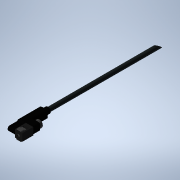
# Autodesk Inventor part: 547859 SMT-8G-PS-24V-E-2,5Q-OE_G
Saved by Autodesk Inventor 2021 (Build 250183000, 183)
## iProperties
Created: 2025-06-24
Part Number: 547859 SMT-8G-PS-24V-E-2,5Q-OE_G
Material: Generic
Catalog Web Link: www.cadenas.de
Description: SMT_G-Proximity switch
Vendor: FESTO
Document SubType Name: Modeling
Designer: psAdmin
Manufacturer: FESTO
Mass: 1.34939 g
Surface Area: 14.7047 cm^2
Volume: 1.34939 cm^3
Density: 1 g/cm^3
Appearance: PSOLRGB-51-51-51
Category: PARTsolutions
Company: FESTO
Title: 547859 SMT-8G-PS-24V-E-2,5Q-OE_G
Author: Cadenas PARTsolutions
Comments: Proximity switch
PSOL_IDENT_0: {$CADENAS_DATA/23d-libs/festo/parts/s/smt/parts/smt_g.prj},204 {VTYP=3D},{NB=547859 SMT-8G-PS-24V-E-
PSOL_IDENT_1: 2,5Q-OE_G},{LINA=547859 SMT-8G-PS-24V-E-2,5Q-OE_G},{NN=SMT_G},{DATE=12.11.2024 13:21:11},{GEOMDATE=3
PSOL_IDENT_2: 0.08.2023 07:21:55},{VERSION=},{LINEID=650},{WBVAR=},{WBNUMERIC=}  {NB=547859 SMT-8G-PS-24V-E-2,5Q-O
PSOL_IDENT_3: E_G},{LINA=547859 SMT-8G-PS-24V-E-2,5Q-OE_G},{KT=DUMMY},{TNR=547859},{TYP=SMT-8G-PS-24V-E-2,5Q-OE},{
PSOL_IDENT_4: VERS=23.000},{AT=OE},{LL=80.000}
NB: 547859 SMT-8G-PS-24V-E-2,5Q-OE_G
NN: SMT_G
NT: Proximity switch
NBSYN: $TNR. $TYP._G
LINA: 547859 SMT-8G-PS-24V-E-2,5Q-OE_G
CATALOG: Festo
TNR: 547859
TYP: SMT-8G-PS-24V-E-2,5Q-OE
VERS: 23
AT: OE
LL: 80
SUPPLIER: FESTO
ARTICLENO: 547859 SMT-8G-PS-24V-E-2,5Q-OE_G
BOMINFO: 547859 SMT-8G-PS-24V-E-2,5Q-OE_G
CREATOR: CADENAS GmbH
Autodesk Inventor part; units mm, degrees
sketch "Sketch_1" plane through (0, 0, 0) normal (0, 0, 1) x (1, 0, 0)
  arc A0 (-2.5, -2.055655) -> (-2.291667, -2.341307) centre (-2.2, -2.055655) ccw
  arc A1 (-2.291667, -2.341307) -> (2.291667, -2.341307) centre (0, 4.8) ccw
  arc A2 (2.291667, -2.341307) -> (2.5, -2.055655) centre (2.2, -2.055655) ccw
  line L0 (2.5, -2.055655) -> (2.5, 2.055655)
  arc A3 (2.5, 2.055655) -> (2.291667, 2.341307) centre (2.2, 2.055655) ccw
  arc A4 (2.291667, 2.341307) -> (-2.291667, 2.341307) centre (0, -4.8) ccw
  arc A5 (-2.291667, 2.341307) -> (-2.5, 2.055655) centre (-2.2, 2.055655) ccw
  line L1 (-2.5, 2.055655) -> (-2.5, -2.055655)
  constraints: 12 point on circle, 6 centre point, 4 end point
extrude "Extrusion1" add sketch "Sketch_1" along normal blind 22.2
sketch "Sketch_2" plane through (0, 0, 0) normal (1, 0, 0) x (0, 1, 0)
  line L0 (-3, 23.2) -> (-3, 14.3)
  line L1 (-3, 14.3) -> (-1.5, 15.8)
  line L2 (-1.5, 15.8) -> (-1.5, 21)
  arc A0 (-0.3, 22.2) -> (-1.5, 21) centre (-0.3, 21) ccw
  line L3 (-0.3, 22.2) -> (0.3, 22.2)
  arc A1 (1.5, 21) -> (0.3, 22.2) centre (0.3, 21) ccw
  line L4 (1.5, 21) -> (1.5, 15.8)
  line L5 (1.5, 15.8) -> (3, 14.3)
  line L6 (3, 14.3) -> (3, 23.2)
  line L7 (3, 23.2) -> (-3, 23.2)
  constraints: 16 end point, 4 point on circle, 2 centre point
extrude "Extrusion2" cut sketch "Sketch_2" along normal mid plane 5
sketch "Sketch_3" plane through (0, 0, 14.8) normal (0, 0, 1) x (1, 0, 0)
  line L0 (0, -2.5) -> (5, -2.5)
  arc A0 (5, -2.5) -> (7.015716, -2.224049) centre (5, 5) ccw
  arc A1 (7.015716, -2.224049) -> (7.224049, -2.015716) centre (6.935087, -1.935087) ccw
  arc A2 (7.224049, -2.015716) -> (7.224049, 2.015716) centre (0, 0) ccw
  arc A3 (7.224049, 2.015716) -> (7.015716, 2.224049) centre (6.935087, 1.935087) ccw
  arc A4 (7.015716, 2.224049) -> (5, 2.5) centre (5, -5) ccw
  line L1 (5, 2.5) -> (0, 2.5)
  line L2 (0, 2.5) -> (0, -2.5)
  constraints: 10 point on circle, 6 end point, 5 centre point
extrude "Extrusion3" add sketch "Sketch_3" against normal blind 4.8
sketch "Sketch_5" plane through (0, 0, 0) normal (0, 1, 0) x (-1, 0, 0)
  line L0 (0, -2.8) -> (0, 1)
  line L1 (0, 1) -> (2.3, 1)
  line L2 (2.3, 1) -> (2.3, 0)
  line L3 (2.3, 0) -> (2.2, 0)
  arc A0 (2.2, 0) -> (2, -0.2) centre (2.2, -0.2) ccw
  line L4 (2, -0.2) -> (2, -2.6)
  arc A1 (1.8, -2.8) -> (2, -2.6) centre (1.8, -2.6) ccw
  line L5 (1.8, -2.8) -> (0, -2.8)
  line L6 (0, -2.8) -> (0, 1)
  constraints: 14 end point, 4 point on circle, 2 centre point
revolve "Revolution1" add sketch "Sketch_5" angle 360 about axis through (0, 0, -2.8) along (0, 0, -1)
sketch "Sketch_28" plane through (0, 0, 0) normal (0, 1, 0) x (-1, 0, 0)
  circle A0 centre (0, 11.4) radius 1.55
  constraints: 1 centre point
extrude "Extrusion4" add sketch "Sketch_28" along normal mid plane 5.4
sketch "Sketch_29" plane through (0, 0, 0) normal (0, 1, 0) x (-1, 0, 0)
  circle A0 centre (0, 18.8) radius 1
  constraints: 1 centre point
extrude "Extrusion5" add sketch "Sketch_29" against normal blind 1.52
sketch "Sketch_6" plane through (0, 0, 0) normal (0, 1, 0) x (-1, 0, 0)
  line L0 (-2.5, 22.3) -> (-3.5, 22.3)
  line L1 (-3.5, 22.3) -> (-3.5, 17)
  line L2 (-3.5, 17) -> (-6.5, 17)
  line L3 (-6.5, 17) -> (-6.5, 22.3)
  line L4 (-6.5, 22.3) -> (-7.5, 22.3)
  line L5 (-7.5, 22.3) -> (-7.5, 14.8)
  line L6 (-7.5, 14.8) -> (-2.5, 14.8)
  line L7 (-2.5, 14.8) -> (-2.5, 22.3)
  constraints: 16 end point
extrude "Extrusion6" add sketch "Sketch_6" along normal mid plane 4.98
sketch "Sketch_7" plane through (5, 0, 0) normal (1, 0, 0) x (0, 0, -1)
  line L0 (-22.3, 2.95) -> (-22.3, -2.95)
  arc A0 (-22.3, -2.95) -> (-22.1, -3.15) centre (-22.1, -2.95) ccw
  line L1 (-22.1, -3.15) -> (-20, -3.15)
  arc A1 (-20, -3.15) -> (-19.8, -2.95) centre (-20, -2.95) ccw
  line L2 (-19.8, -2.95) -> (-19.8, -2.7)
  arc A2 (-19.6, -2.5) -> (-19.8, -2.7) centre (-19.6, -2.7) ccw
  line L3 (-19.6, -2.5) -> (-18.5, -2.5)
  arc A3 (-18.5, -2.5) -> (-18.3, -2.3) centre (-18.5, -2.3) ccw
  line L4 (-18.3, -2.3) -> (-18.3, 2.3)
  arc A4 (-18.3, 2.3) -> (-18.5, 2.5) centre (-18.5, 2.3) ccw
  line L5 (-18.5, 2.5) -> (-19.6, 2.5)
  arc A5 (-19.8, 2.7) -> (-19.6, 2.5) centre (-19.6, 2.7) ccw
  line L6 (-19.8, 2.7) -> (-19.8, 2.95)
  arc A6 (-19.8, 2.95) -> (-20, 3.15) centre (-20, 2.95) ccw
  line L7 (-20, 3.15) -> (-22.1, 3.15)
  arc A7 (-22.1, 3.15) -> (-22.3, 2.95) centre (-22.1, 2.95) ccw
  constraints: 16 end point, 16 point on circle, 8 centre point
extrude "Extrusion7" add sketch "Sketch_7" along normal mid plane 3
sketch "Sketch_4" plane through (0, 0, 0) normal (0, 1, 0) x (-1, 0, 0)
  line L0 (-5, 22.3) -> (-5, 10)
  line L1 (-5, 10) -> (-6.4, 10)
  line L2 (-6.4, 10) -> (-6.05, 10.35)
  line L3 (-6.05, 10.35) -> (-6.05, 18.3)
  line L4 (-6.05, 18.3) -> (-6.1, 18.3)
  line L5 (-6.1, 18.3) -> (-5.8645, 18.5355)
  line L6 (-5.8645, 18.5355) -> (-5.8645, 22.3)
  line L7 (-5.8645, 22.3) -> (-5, 22.3)
  line L8 (-5, 22.3) -> (-5, 10)
  constraints: 18 end point
revolve "Revolution2" cut sketch "Sketch_4" angle 360 about axis through (5, 0, 22.3) along (0, 0, 1)
thread "Thread1" size "M2x0.25" class "6H" standard "ISO Metric profile" full length
sketch "Sketch_8" plane through (0, 0, 0) normal (0, 1, 0) x (-1, 0, 0)
  line L0 (-5, 22) -> (-5, 8)
  line L1 (-5, 8) -> (-7.2, 8)
  arc A0 (-7.4, 8.2) -> (-7.2, 8) centre (-7.2, 8.2) ccw
  line L2 (-7.4, 8.2) -> (-7.4, 10)
  line L3 (-7.4, 10) -> (-6.05, 10)
  line L4 (-6.05, 10) -> (-6.05, 15.95)
  line L5 (-6.05, 15.95) -> (-6, 16)
  line L6 (-6, 16) -> (-6, 21.8465)
  line L7 (-6, 21.8465) -> (-5.8465, 22)
  line L8 (-5.8465, 22) -> (-5, 22)
  line L9 (-5, 22) -> (-5, 8)
  constraints: 20 end point, 2 point on circle, 1 centre point
revolve "Revolution3" add sketch "Sketch_8" angle 360 about axis through (5, 0, 22) along (0, 0, 1)
sketch "Sketch_9" plane through (0, 0, 8) normal (0, 0, 1) x (1, 0, 0)
  line L0 (4.25, -0.433013) -> (5, -0.866025)
  line L1 (5, -0.866025) -> (5.75, -0.433013)
  line L2 (5.75, -0.433013) -> (5.75, 0.433013)
  line L3 (5.75, 0.433013) -> (5, 0.866025)
  line L4 (5, 0.866025) -> (4.25, 0.433013)
  line L5 (4.25, 0.433013) -> (4.25, -0.433013)
  constraints: 12 end point
extrude "Extrusion8" cut sketch "Sketch_9" along normal blind 1
sketch "Sketch_10" plane through (0, 0, 0) normal (1, 0, 0) x (0, 1, 0)
  line L0 (0, -80) -> (0, -2.8)
  line L1 (0, -2.8) -> (1.45, -2.8)
  line L2 (1.45, -2.8) -> (1.45, -80)
  line L3 (1.45, -80) -> (0, -80)
  line L4 (0, -80) -> (0, -2.8)
  constraints: 10 end point
revolve "Revolution4" add sketch "Sketch_10" angle 360 about axis through (0, 0, -80) along (0, 0, -1)
sketch "Sketch_27" plane through (0, 0, 0) normal (1, 0, 0) x (0, 1, 0)
  line L0 (1.45, -74.977053) -> (-1.45, -80)
  line L1 (-1.45, -80) -> (1.45, -80)
  line L2 (1.45, -80) -> (1.45, -74.977053)
  constraints: 6 end point
extrude "Extrusion9" cut sketch "Sketch_27" along normal mid plane 2.9
ref_plane "DUMMY_XY" through (0, 0, 0) normal (0, 0, -1) x (1, 0, 0)
ref_plane "DUMMY_YZ" through (0, 0, 0) normal (1, 0, 0) x (0, -1, 0)
ref_plane "DUMMY_ZX" through (0, 0, 0) normal (0, -1, 0) x (0, 0, -1)
ref_plane "KTN1_XY" through (0, 0, -68) normal (0, 0, 1) x (0, 1, 0)
ref_plane "KTN1_YZ" through (0, 0, -68) normal (0, 1, 0) x (-1, 0, 0)
ref_plane "KTN1_ZX" through (0, 0, -68) normal (-1, 0, 0) x (0, 0, 1)
ref_plane "KTN2_XY" through (0, 0, -9.8) normal (0, 0, -1) x (0, 1, 0)
ref_plane "KTN2_YZ" through (0, 0, -9.8) normal (0, 1, 0) x (1, 0, 0)
ref_plane "KTN2_ZX" through (0, 0, -9.8) normal (1, 0, 0) x (0, 0, -1)
body "Solid1"
